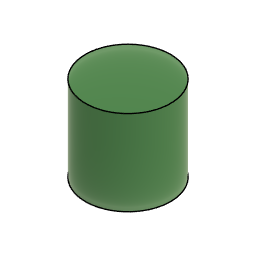
PE1-PE7 - PCB Enclosure Subassembly (Autodesk Fusion 360 archive; units mm, degrees)
design "Traceline Dummy"
Autodesk Fusion 360 part; units mm, degrees
note: some values were not read from the file. Chosen so that the rebuilt part matches the saved one: which bodies a step acts on; which face or edge a step refers to; the layout of a text. Set by a fixed rule: which sketch regions a step uses.
sketch "Sketch1" plane through (0, 0, 0) normal (0, 0, 1) x (1, 0, 0)
  circle A0 centre (0, 0) radius 0.05
  dimension "d1" = 0.1
  constraint coincident A0.centre origin
  measures "d1" diameter of A0
extrude "Extrude1" add sketch "Sketch1" along normal blind 0.1

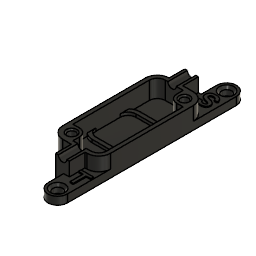
design "PE3 - PCB Case"
Autodesk Fusion 360 part; units mm, degrees
sketch "Sketch1" plane through (0, 0, 0) normal (0, 0, 1) x (1, 0, 0)
  line L0 (6.2013, 10.25) -> (-6.2012, 10.25)
  line L1 (-10.25, 6.2013) -> (-10.25, -6.2012)
  line L2 (-6.2012, -10.25) -> (6.2013, -10.25)
  line L3 (10.25, -6.2012) -> (10.25, 6.2012)
  line L4 (10.25, 10.25) -> (-10.25, -10.25) construction
  line L5 (-10.25, 10.25) -> (10.25, -10.25) construction
  arc A0 (-6.2012, 10.25) -> (-10.25, 6.2013) centre (-6.2013, 6.2013) ccw
  arc A1 (10.25, 6.2012) -> (6.2013, 10.25) centre (6.2012, 6.2012) ccw
  arc A2 (-10.25, -6.2012) -> (-6.2012, -10.25) centre (-6.2013, -6.2013) ccw
  arc A3 (6.2013, -10.25) -> (10.25, -6.2012) centre (6.2013, -6.2013) ccw
  line L6 (-12.25, 6.2013) -> (-12.25, -6.2013)
  arc A4 (-12.25, -6.2012) -> (-6.2012, -12.25) centre (-6.2013, -6.2013) ccw
  line L7 (-6.2012, -12.25) -> (6.2013, -12.25)
  arc A5 (6.2013, -12.25) -> (12.25, -6.2012) centre (6.2013, -6.2013) ccw
  line L8 (12.25, -6.2012) -> (12.25, 6.2012)
  arc A6 (12.25, 6.2012) -> (6.2013, 12.25) centre (6.2012, 6.2012) ccw
  line L9 (6.2013, 12.25) -> (-6.2012, 12.25)
  arc A7 (-6.2012, 12.25) -> (-12.25, 6.2013) centre (-6.2013, 6.2013) ccw
  dimension "d1" = 20.5
  dimension "d2" = 20.5
  dimension "d3" = 4.0488
  dimension "d4" = 4.0488
  dimension "d5" = 4.0488
  dimension "d6" = 4.0488
  dimension "d7" = 2
  constraint horizontal L0
  constraint perpendicular L0 L1
  constraint parallel L0 L2
  constraint parallel L1 L3
  constraint coincident L4 origin
  constraint coincident L5 origin
  constraint coincident L5.start L0
  constraint coincident L5.start L1
  constraint tangent L0 A0
  constraint tangent L1 A0
  constraint coincident L4.start L0
  constraint coincident L4.start L3
  constraint tangent L0 A1
  constraint tangent L3 A1
  constraint coincident L4.end L2
  constraint coincident L4.end L1
  constraint tangent L2 A2
  constraint tangent L1 A2
  constraint coincident L5.end L3
  constraint coincident L5.end L2
  constraint tangent L3 A3
  constraint tangent L2 A3
  measures "d1" distance of L4.start L5.start
  measures "d2" distance of L4.start L5.end
  measures "d3" radius of A0
  measures "d4" radius of A1
  measures "d5" radius of A2
  measures "d6" radius of A3
extrude "Extrude1" add sketch "Sketch1" along normal blind 6 contours L0 L1 L2 L3 A0 A1 A2 A3 | L6 A4 L7 A5 L8 A6 L9 A7
extrude "Extrude2" add sketch "Sketch1" along normal blind 1.5 from surface at 6
sketch "Sketch10" plane through (0, 0, 0) normal (0, 0, 1) x (1, 0, 0)
  line L0 (7.2501, -43.2789) -> (7.2501, 43.2211) construction
  line L1 (7.2501, -0.0289) -> (8.1135, -0.0289) construction
  circle A0 centre (7.2501, 43.2211) radius 2.5
  circle A1 centre (7.2501, -43.2789) radius 2.5
  arc A2 (2.2502, -43.2493) -> (12.25, -43.25) centre (7.2501, -43.2789) ccw
  arc A3 (12.25, 43.1922) -> (2.2502, 43.1914) centre (7.2501, 43.2211) ccw
  line L2 (2.2502, 43.1914) -> (2.2502, -43.3086)
  line L3 (12.25, -43.25) -> (12.25, 43.25)
  dimension "d42" = 86.5
  dimension "d43" = 5
  dimension "d44" = 5
  dimension "d45" = 10
  dimension "d46" = 10
  dimension "d134" = 0.0289
  dimension "d135" = 7.2501
  dimension "d136" = 0.8634
  constraint midpoint L0 L1.start
  constraint perpendicular L0 L1
  constraint coincident L0.end A0.centre
  constraint coincident L0.start A1.centre
  constraint concentric A1 A2
  constraint concentric A0 A3
  constraint parallel L0 L2
  constraint coincident A2 L2.end
  constraint coincident L2 A2.start
  constraint vertical L3
  constraint coincident L3 A3.start
  constraint coincident A3 L3.end
  constraint parallel L0 L3
  constraint equal L0 L2
  constraint equal L0 L3
  measures "d42" distance of L0.start L0.end
  measures "d43" diameter of A0
  measures "d44" diameter of A1
  measures "d45" diameter of A2
  measures "d46" diameter of A3
  measures "d134" distance of origin L1
  measures "d135" distance of origin L0
  measures "d136" distance of L0 L1.end
extrude "Extrude10" add sketch "Sketch10" along normal blind 4
chamfer "Chamfer1" distance 1.25 angle 45 2 edges at (6.346, -45.6097, 4) (6.346, 40.8903, 4)
sketch "Sketch12" plane through (0, 0, 0) normal (0, 0, -1) x (1, 0, 0)
  circle A0 centre (7.2501, 43.2789) radius 2.5
  circle A1 centre (7.2501, -43.2211) radius 2.5
  line L0 (2.2502, 12.25) -> (-6.2012, 12.25)
  arc A2 (-6.2013, 12.25) -> (-12.25, 6.2012) centre (-6.2013, 6.2013) ccw
  line L1 (-12.25, 6.2012) -> (-12.25, -6.2013)
  arc A3 (-12.25, -6.2013) -> (-6.2012, -12.25) centre (-6.2013, -6.2013) ccw
  line L2 (2.2502, -12.25) -> (2.2502, -43.1914)
  arc A4 (2.2502, -43.1914) -> (12.25, -43.25) centre (7.2501, -43.2211) ccw
  line L3 (12.25, -43.25) -> (12.25, 43.25)
  arc A5 (12.25, 43.25) -> (2.2502, 43.3086) centre (7.2501, 43.2789) ccw
  line L4 (10.25, -21.2012) -> (10.25, 21.2013)
  arc A6 (-6.2013, 25.25) -> (-10.25, 21.2013) centre (-6.2013, 21.2013) ccw
  arc A7 (-12.25, -21.2012) -> (-6.2013, -27.25) centre (-6.2013, -21.2012) ccw
  arc A8 (6.2013, -25.25) -> (10.25, -21.2012) centre (6.2013, -21.2012) ccw
  line L5 (-10.25, 25.25) -> (10.25, -25.25) construction
  line L6 (10.25, 25.25) -> (-10.25, -25.25) construction
  line L7 (-12.25, 21.2012) -> (-12.25, -21.2012)
  line L8 (-10.25, 21.2013) -> (-10.25, -21.2012)
  arc A9 (12.25, 21.2013) -> (6.2013, 27.25) centre (6.2012, 21.2013) ccw
  arc A10 (-6.2012, 27.25) -> (-12.25, 21.2012) centre (-6.2013, 21.2013) ccw
  line L9 (-6.2013, -25.25) -> (6.2013, -25.25)
  line L10 (6.2012, 25.25) -> (-6.2013, 25.25)
  line L11 (12.25, -21.2012) -> (12.25, 21.2013)
  arc A11 (10.25, 21.2013) -> (6.2012, 25.25) centre (6.2012, 21.2013) ccw
  arc A12 (-10.25, -21.2012) -> (-6.2013, -25.25) centre (-6.2013, -21.2012) ccw
  arc A13 (6.2012, -27.25) -> (12.25, -21.2012) centre (6.2013, -21.2012) ccw
  line L12 (-6.2013, -27.25) -> (6.2012, -27.25)
  line L13 (6.2013, 27.25) -> (-6.2012, 27.25)
  line L14 (-6.2012, -12.25) -> (2.2502, -12.25)
  line L15 (2.2502, 43.3086) -> (2.2502, 12.25)
  dimension "d77" = 2
  dimension "d78" = 20.5
  dimension "d79" = 50.5
  dimension "d80" = 4.0488
  dimension "d81" = 4.0488
  dimension "d82" = 4.0488
  dimension "d83" = 4.0488
  constraint horizontal L10
  constraint perpendicular L8 L10
  constraint parallel L9 L10
  constraint parallel L4 L8
  constraint coincident origin L6
  constraint coincident origin L5
  constraint coincident L5.start L10
  constraint coincident L5.start L8
  constraint tangent A6 L10
  constraint tangent A6 L8
  constraint coincident L6.start L10
  constraint coincident L6.start L4
  constraint tangent L10 A11
  constraint tangent L4 A11
  constraint coincident L6.end L9
  constraint coincident L6.end L8
  constraint tangent L9 A12
  constraint tangent L8 A12
  constraint coincident L5.end L4
  constraint coincident L5.end L9
  constraint tangent L4 A8
  constraint tangent A8 L9
  measures "d78" distance of L5.start L6.start
  measures "d79" distance of L5.end L6.start
  measures "d80" radius of A6
  measures "d81" radius of A11
  measures "d82" radius of A12
  measures "d83" radius of A8
extrude "Extrude13" cut 1 faces at (-3.4167, 2.0671, 6) along direction (0, 0, -1) blind 1
extrude "Extrude14" add sketch "Sketch12" against normal blind 11 contours L2 L3 L4 A8 A9 L9 L10 L11 A11 A13 L12 L13 L15 | A2 A6 L7 L8 A10 L10 L13 L15 | A2 L1 A3 L7 L8 | A3 L2 A7 L7 L8 L9 A12 L12
extrude "Extrude15" add sketch "Sketch12" against normal blind 4 contours L0 A2 A6 L8 L10 L15 | A3 L2 L8 L9 A12 L14
sketch "Sketch13" plane through (0, -27.25, 0) normal (0, -1, 0) x (1, 0, 0)
  line L0 (2.2502, 0) -> (2.2502, 4)
  line L1 (2.2502, 4) -> (6.2013, 4)
  line L2 (6.2013, 4) -> (6.2013, 11)
  line L3 (6.2013, 11) -> (-6.2012, 11)
  line L4 (-6.2012, 11) -> (-6.2012, 0)
  line L5 (-6.2012, 0) -> (2.2502, 0)
  line L6 (-1.8, 0) -> (5.2012, 0)
  line L7 (5.2012, 11) -> (5.2012, 0)
  line L8 (6.2012, 4) -> (3.0821, 4)
  line L9 (-1.8, 11) -> (-1.8, -1.0165)
  line L10 (-1.8, 0) -> (5.2012, 0)
  line L11 (-1.8, -1.0165) -> (-1.8, 0)
  line L12 (3.85, 11) -> (5.2012, 11)
  line L13 (-0.45, 11) -> (-1.8, 11)
  arc A0 (-0.45, 11) -> (3.85, 11) centre (1.7, 11) ccw
  point P0 (1.7, 11)
  dimension "d89" = 7
  dimension "d90" = 4.3
  constraint horizontal L10
  constraint horizontal L8
  constraint coincident P0 A0.centre
  constraint coincident L6.end L7.end
  constraint perpendicular L6 L7
  constraint perpendicular L10 L11
  constraint coincident L5 L6.start
  constraint perpendicular L7 L12
  constraint perpendicular L9 L13
  measures "d89" distance of L9.end L8.end
  measures "d90" diameter of A0
sketch "Sketch14" plane through (0, 27.25, 0) normal (0, 1, 0) x (-1, 0, 0)
  line L0 (-2.2502, 4) -> (-2.2502, 0)
  line L1 (-2.2502, 0) -> (6.2013, 0)
  line L2 (6.2013, 0) -> (6.2013, 11)
  line L3 (6.2013, 11) -> (-6.2012, 11)
  line L4 (-6.2012, 11) -> (-6.2012, 4)
  line L5 (-6.2012, 4) -> (-2.2502, 4)
  line L6 (-6.2013, 0) -> (-6.2013, 4)
  line L7 (-0.8, 15) -> (-0.8, 4)
  line L8 (-6.2013, 0) -> (6.2012, 0)
  line L9 (-0.8, 15) -> (6.2012, 15)
  line L10 (6.2012, 4) -> (6.2, 4)
  line L11 (6.2012, 15) -> (6.2012, 0)
  circle A0 centre (2.7, 11) radius 2.15
  line L12 (-0.8, 4) -> (-6.2013, 4)
  line L13 (-6.2013, 0) -> (6.2012, 0)
  point P0 (2.7, 11)
  dimension "d91" = 7
  dimension "d92" = 4.3
  dimension "d137" = 12.4012
  dimension "d138" = 7
  dimension "d139" = 11
  dimension "d140" = 0.0012
  dimension "d141" = 3.5
  constraint horizontal L13
  constraint horizontal L10
  constraint collinear L10 L12
  constraint coincident P0 A0.centre
  constraint coincident L8.end L11.end
  constraint perpendicular L8 L11
  constraint coincident L6.start L8.start
  constraint perpendicular L6 L12
  constraint coincident L4.end L6.end
  constraint perpendicular L7 L12
  constraint equal L0 L6
  constraint coincident L10.start L11
  constraint perpendicular L7 L9
  constraint coincident L1 origin
  measures "d91" distance of L7.end L10.end
  measures "d92" diameter of A0
  measures "d137" distance of L4 L10.end
  measures "d138" distance of L5 P0
  measures "d139" distance of L10.start L9
  measures "d140" distance of L10.end L11
  measures "d141" distance of P0 L7
extrude "Extrude16" add sketch "Sketch13" along normal blind 8 contours L0 L1 L3 L5 L6 L7 L8 L9 L10 L12 L13 A0
extrude "Extrude17" add sketch "Sketch13" along normal blind 8 contours L0 L1 L3 L5 L6 L7 L8 L9 L10 L12 L13 A0
extrude "Extrude18" add sketch "Sketch14" along normal blind 8 contours L0 L1 L2 L3 L7 L8 L11 A0 L12 L13
extrude "Extrude19" cut 1 faces at (-2.4382, 27.25, 10.3329) along direction (0, -1, 0) blind 5
extrude "Extrude20" cut 1 faces at (1.9618, -27.25, 10.3329) along direction (0, 1, 0) blind 4
sketch "Sketch15" plane through (0, 0, 4) normal (0, 0, 1) x (-1, 0, 0)
  line L0 (-10.25, 21.2013) -> (-10.25, 10.6951)
  arc A0 (-6.2013, 12.25) -> (-10.25, 10.6951) centre (-6.2013, 6.2013) ccw
  line L1 (-6.2013, 12.25) -> (6.2013, 12.25)
  arc A1 (10.25, 10.6951) -> (6.2012, 12.25) centre (6.2013, 6.2013) ccw
  line L2 (10.25, 10.6951) -> (10.25, 21.2013)
  arc A2 (10.25, 21.2013) -> (6.2013, 25.25) centre (6.2013, 21.2013) ccw
  line L3 (6.2013, 25.25) -> (-6.2012, 25.25)
  arc A3 (-6.2012, 25.25) -> (-10.25, 21.2013) centre (-6.2012, 21.2013) ccw
  circle A4 centre (6.9428, 21.9428) radius 2
  line L4 (8.8794, 25.9428) -> (2.9428, 25.9428)
  line L5 (2.9428, 25.9428) -> (2.9428, 21.9428)
  line L6 (6.9428, 17.9428) -> (10.9428, 17.9428)
  line L7 (10.9428, 17.9428) -> (10.9428, 23.8794)
  arc A5 (2.9428, 21.9428) -> (6.9428, 17.9428) centre (6.9428, 21.9428) ccw
  line L8 (10.9428, 17.9428) -> (10.9428, 23.8794)
  line L9 (8.8794, 25.9428) -> (2.9428, 25.9428)
  line L10 (2.9428, 25.9428) -> (2.9428, 21.9428)
  line L11 (6.9428, 17.9428) -> (10.9428, 17.9428)
  arc A6 (2.9428, 21.9428) -> (6.9428, 17.9428) centre (6.9428, 21.9428) ccw
  circle A7 centre (6.9428, 21.9428) radius 2
  line L12 (-1.75, 0) -> (-22.5, 0) construction
  line L13 (0, -2.5) -> (0, -20) construction
  line L14 (-8.0247, -25.9428) -> (-2.9428, -25.9428)
  line L15 (-2.9428, -25.9428) -> (-2.9428, -21.9428)
  arc A8 (-2.9428, -21.9428) -> (-6.9428, -17.9428) centre (-6.9428, -21.9428) ccw
  line L16 (-10.9428, -17.9428) -> (-10.9428, -23.0247)
  line L17 (-6.9428, -17.9428) -> (-10.9428, -17.9428)
  circle A9 centre (-6.9428, -21.9428) radius 2
  line L18 (-8.0247, -25.9428) -> (-10.9428, -23.0247)
  line L19 (-8.0247, -25.9428) -> (-3.8978, -25.9428) construction
  line L20 (10.9428, 23.8794) -> (8.8794, 25.9428)
  point P0 (6.9428, 21.9428)
  dimension "d106" = 4
  dimension "d109" = 4
  dimension "d114" = 4
  dimension "d115" = 4
  dimension "d116" = 135
  dimension "d142" = 17.9428
  dimension "d143" = 25.9428
  dimension "d144" = 23.0247
  dimension "d145" = 5.8857
  dimension "d149" = 23.8794
  dimension "d150" = 5.9366
  dimension "d151" = 17.9428
  dimension "d152" = 8
  constraint horizontal L4
  constraint perpendicular L4 L5
  constraint parallel L4 L6
  constraint parallel L5 L7
  constraint tangent L5 A5
  constraint tangent L6 A5
  constraint horizontal L9
  constraint perpendicular L9 L10
  constraint parallel L9 L11
  constraint parallel L8 L10
  constraint tangent L10 A6
  constraint tangent L11 A6
  constraint horizontal L19
  constraint tangent A8 L17
  constraint tangent L15 A8
  constraint concentric A8 A9
  constraint concentric A5 A7
  constraint equal A5 A8
  constraint midpoint A5 A6
  constraint equal L5 L10
  constraint equal L5 L11
  constraint equal L5 L15
  constraint equal L5 L17
  constraint perpendicular L16 L17
  constraint equal L18 L19
  constraint equal A4 A9
  constraint concentric A4 A5
  constraint coincident P0 A4.centre
  measures "d106" diameter of A4
  measures "d109" radius of A5
  measures "d114" diameter of A7
  measures "d115" radius of A6
  measures "d116" angle of L18 L19
  measures "d142" distance of L12 L17
  measures "d143" distance of L12 L19
  measures "d144" distance of L12 L16.end
  measures "d145" distance of L5 L15
  measures "d149" distance of L12 L7.end
  measures "d150" distance of L5 L4.start
  measures "d151" distance of L6 L12
  measures "d152" distance of L5 L7
extrude "Extrude21" add sketch "Sketch15" along normal blind 7 contours L2 A2 L3 L5 L6 A5 L10 L11 A6 | L14 L15 A8 L16 L17 L18
chamfer "Chamfer5" distance 0.7 angle 45 2 edges at (8.8075, 21.2196, 11) (-5.0782, -22.6661, 11)
extrude "Extrude24" cut 2 faces at (3.0992, -19.4386, 4) (-3.0992, 19.4386, 4) along direction (0, 0, -1) blind 2
extrude "Extrude25" cut 1 faces at (-3.4167, 2.0671, 5) along direction (0, 0, -1) blind 3
sketch "Sketch16" plane through (0, 0, 4) normal (0, 0, 1) x (-1, 0, 0)
  arc A0 (-12.25, -21.2012) -> (-6.2012, -27.25) centre (-6.2013, -21.2012) ccw
  line L0 (-12.25, -21.2012) -> (-12.25, -43.25)
  arc A1 (-12.25, -43.25) -> (-2.2502, -43.1914) centre (-7.2501, -43.2211) ccw
  line L1 (-2.2502, -43.1914) -> (-2.2502, -35.25)
  line L2 (-2.2502, -35.25) -> (-0.8, -35.25)
  line L3 (-0.8, -35.25) -> (-0.8, -27.25)
  line L4 (-10.7579, -32.3932) -> (-6.9514, -32.3932) construction
  line L5 (-6.9514, -32.3932) -> (-6.9514, -27.9161) construction
  line L6 (-6.9514, -27.9161) -> (-10.7579, -27.9161) construction
  line L7 (-10.7579, -27.9161) -> (-10.7579, -32.3932) construction
  line L8 (-0.8, -27.25) -> (-6.2012, -27.25)
  circle A2 centre (-7.2501, -43.2211) radius 3.75
  dimension "d124" = 8
  dimension "d153" = 5.2986
  dimension "d154" = 15.3339
  dimension "d155" = 3.8065
  dimension "d156" = 4.4771
  text T0 "S" font "Arial" height 8 bold align left top in box 3.8065 x 4.4771 at (-10.7579, -32.3932) x (1, 0) y (0, 1) spacing 1 by line height
  measures "d153" distance of L0 L5
  measures "d154" distance of L0.end L6
  measures "d155" distance of L5 L7
  measures "d156" distance of L4 L6
extrude "Extrude26" add sketch "Sketch16" along normal blind 0.5 text T0
sketch "Sketch17" plane through (0, 0, 4) normal (0, 0, 1) x (-1, 0, 0)
  circle A0 centre (-7.2501, 43.2789) radius 3.75
  line L0 (-5.2012, 27.25) -> (-5.2012, 35.25)
  line L1 (-5.2012, 35.25) -> (-2.2502, 35.25)
  line L2 (-2.2502, 35.25) -> (-2.2502, 43.3086)
  arc A1 (-2.2502, 43.3086) -> (-12.25, 43.25) centre (-7.2501, 43.2789) ccw
  line L3 (-12.25, 43.25) -> (-12.25, 21.2013)
  arc A2 (-6.2013, 27.25) -> (-12.25, 21.2013) centre (-6.2012, 21.2013) ccw
  line L4 (-6.2013, 27.25) -> (-5.2012, 27.25)
  line L5 (-5.3111, 31.9604) -> (-9.1175, 31.9604) construction
  line L6 (-9.1175, 31.9604) -> (-9.1175, 27.4833) construction
  line L7 (-9.1175, 27.4833) -> (-5.3111, 27.4833) construction
  line L8 (-5.3111, 27.4833) -> (-5.3111, 31.9604) construction
  dimension "d127" = 8
  dimension "d157" = 6.9389
  dimension "d158" = 6.282
  dimension "d159" = 4.4771
  dimension "d160" = 3.8065
  text T0 "T" font "Arial" height 8 bold align left top in box 3.8065 x 4.4771 at (-5.3111, 31.9604) x (-1, 0) y (0, -1) spacing 1 by line height
  constraint vertical L8
  measures "d157" distance of L3 L8
  measures "d158" distance of L3.end L7
  measures "d159" distance of L5 L7
  measures "d160" distance of L6 L8
extrude "Extrude27" add sketch "Sketch17" along normal blind 0.5 text T0
extrude "Extrude28" cut 2 faces at (-2.0671, 10.9167, 7.5) (-2.0671, -11.5833, 7.5) along direction (0, 0, -1) blind 4
equation "d3 = ( 20.5 / 20 * 3.95 ) * 1 mm"
equation "d4 = ( 20.5 / 20 * 3.95 ) * 1 mm"
equation "d5 = ( 20.5 / 20 * 3.95 ) * 1 mm"
equation "d6 = ( 20.5 / 20 * 3.95 ) * 1 mm"
equation "d80 = ( 20.5 / 20 * 3.95 ) * 1 mm"
equation "d81 = ( 20.5 / 20 * 3.95 ) * 1 mm"
equation "d82 = ( 20.5 / 20 * 3.95 ) * 1 mm"
equation "d83 = ( 20.5 / 20 * 3.95 ) * 1 mm"

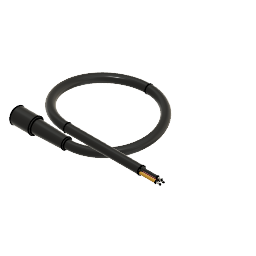
design "PE2 - 3-Pin Male Waterproof Connector (coiled)"
Autodesk Fusion 360 part; units mm, degrees
sketch "Sketch1" plane through (0, 0, 0) normal (1, 0, 0) x (0, 1, 0)
  circle A0 centre (0, 0) radius 3.683
  circle A1 centre (0, 0) radius 3.175
  dimension "d1" = 7.366
  dimension "d2" = 6.35
  constraint coincident A0.centre A1.centre
  constraint concentric A0 A1
  measures "d1" diameter of A0
  measures "d2" diameter of A1
extrude "Extrude1" add sketch "Sketch1" along normal blind 10 contours A0 | A1 makes body 1
extrude "Extrude2" cut sketch "Sketch1" along normal blind 8 contours A1 bodies 1
sketch "Sketch2" plane through (0, 0, 0) normal (0, 1, 0) x (1, 0, 0)
  line L0 (10, 0) -> (10, -3)
  line L1 (10, -3) -> (25, -2.5)
  line L2 (25, -2.5) -> (25, 0)
  line L3 (25, 0) -> (10, 0)
  dimension "d7" = 3
  dimension "d44" = 15
  dimension "d45" = 88.091
  dimension "d46" = 10
  constraint vertical L0
  constraint vertical L2
  constraint perpendicular L0 L3
  constraint horizontal origin L0.start
  measures "d7" distance of L0.start L0.end
  measures "d44" distance of L0 L2
  measures "d45" angle of L0 L1
  measures "d46" distance of origin L0
revolve "Revolve1" add sketch "Sketch2" angle 360 about axis through (1.75, 0, 0) along (1, 0, 0) bodies 1
fillet "Fillet1" radius 0.5 3 edges at (0, -3.4338, -1.3318) (10, -3.4338, -1.3318) (25, -0.904, -2.3308) on bodies 1
sketch "Sketch4" plane through (8, 0, 0) normal (1, 0, 0) x (0, 1, 0)
  line L0 (0, 1.5) -> (-1.299, -0.75) construction
  line L1 (-1.299, -0.75) -> (1.299, -0.75) construction
  line L2 (1.299, -0.75) -> (0, 1.5) construction
  circle A0 centre (0, 1.5) radius 0.5
  circle A1 centre (-1.299, -0.75) radius 0.5
  circle A2 centre (1.299, -0.75) radius 0.5
  dimension "d15" = 1.5
  dimension "d16" = 1
  dimension "d17" = 1
  dimension "d18" = 1
  constraint coincident L0.start L2.end
  constraint coincident L0.end L1.start
  constraint coincident L1.end L2.start
  constraint horizontal L1
  measures "d15" distance of L0.start origin
  measures "d16" diameter of A0
  measures "d17" diameter of A1
  measures "d18" diameter of A2
extrude "Extrude4" add sketch "Sketch4" against normal blind 8 separate body makes body 2 at (2.6667, 0.4975, 1.4502) makes body 3 at (2.6667, 1.7966, -0.7998) makes body 4 at (2.6667, -0.8015, -0.7998)
fillet "Fillet2" radius 0.1 3 edges at (0, -0.4662, 1.6808) (0, 0.8329, -0.5692) (0, -1.7652, -0.5692) on bodies 2 3 4
sketch "Sketch3" plane through (25, 0, 0) normal (1, 0, 0) x (0, 1, 0)
  circle A0 centre (0, 0) radius 1.905
  circle A1 centre (0, 0) radius 2.0164
  dimension "d9" = 3.81
  constraint coincident A0.centre A1.centre
  measures "d9" diameter of A0
sketch "Sketch5" plane through (0, 0, 0) normal (0, 0, 1) x (1, 0, 0)
  arc A0 through (25, 0, 0) (45, 19.9239, 1.7431) (25, 39.8478, 3.4862)
  arc A1 through (25, 39.8478, 3.4862) (5, 19.9239, 5.2293) (25, 0, 6.9725)
  dimension "d42" = 40
  dimension "d47" = 20
  dimension "d48" = 3.4862
  dimension "d49" = 6.9725
sweep "Sweep1" add profiles "Sketch3" path "Sketch5" along A0 A1 section 1 contours A0 bodies 1
extrude "Extrude5" add 1 faces at (25, -0.7992, 7.2336) along direction (1, 0, 0) blind 36.2 on bodies 1 bodies 1
sketch "Sketch6" plane through (61.2, 0, 0) normal (1, 0, 0) x (0, 1, 0)
  line L0 (0, 7.9725) -> (-0.866, 6.4725) construction
  line L1 (-0.866, 6.4725) -> (0.866, 6.4725) construction
  line L2 (0.866, 6.4725) -> (0, 7.9725) construction
  circle A0 centre (0, 7.9725) radius 0.625
  circle A1 centre (0.866, 6.4725) radius 0.625
  circle A2 centre (-0.866, 6.4725) radius 0.625
  circle A3 centre (0, 6.9725) radius 1.905
  point P0 (0, 6.9725)
  dimension "d31" = 1
  dimension "d32" = 1.25
  dimension "d33" = 1.25
  dimension "d34" = 1.25
  constraint coincident L0.start L2.end
  constraint coincident L1.end L2.start
  constraint coincident L0.end L1.start
  constraint coincident P0 A3.centre
  constraint vertical L0.start P0
  measures "d31" distance of L0.start P0
  measures "d32" diameter of A0
  measures "d33" diameter of A1
  measures "d34" diameter of A2
extrude "Extrude6" add sketch "Sketch6" along normal blind 8 separate body contours A0 | A1 | A2 makes body 5 at (63.8667, 0.6219, 7.9102) makes body 6 at (63.8667, -0.2441, 6.4102) makes body 7 at (63.8667, 1.4879, 6.4102)
sketch "Sketch7" plane through (69.2, 0, 0) normal (1, 0, 0) x (0, 1, 0)
  circle A0 centre (0, 7.9725) radius 0.625
  circle A1 centre (0, 7.9725) radius 0.375
  dimension "d43" = 0.75
  constraint concentric A0 A1
  measures "d43" diameter of A1
sketch "Sketch8" plane through (69.2, 0, 0) normal (1, 0, 0) x (0, 1, 0)
  circle A0 centre (0.866, 6.4725) radius 0.625
  circle A1 centre (0.866, 6.4725) radius 0.375
  dimension "d37" = 0.75
  constraint concentric A0 A1
  measures "d37" diameter of A1
sketch "Sketch9" plane through (69.2, 0, 0) normal (1, 0, 0) x (0, 1, 0)
  circle A0 centre (-0.866, 6.4725) radius 0.625
  circle A1 centre (-0.866, 6.4725) radius 0.375
  dimension "d38" = 0.75
  constraint concentric A0 A1
  measures "d38" diameter of A1
extrude "Extrude7" add sketch "Sketch9" sketch "Sketch8" sketch "Sketch7" along normal blind 2 separate body contours A1 of sketch 2 contours A1 of sketch 3 contours A1 makes body 8 at (69.8667, 1.2392, 6.4351) makes body 9 at (69.8667, -0.4929, 6.4351) makes body 10 at (70.5333, -0.3524, 8.1007)

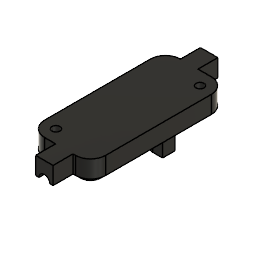
design "PE4 - PCB Case Lid"
Autodesk Fusion 360 part; units mm, degrees
sketch "Sketch1" plane through (0, 0, 0) normal (0, 0, 1) x (1, 0, 0)
  line L0 (6.2013, 11.75) -> (-6.2012, 11.75)
  line L1 (10.25, 10.25) -> (-10.25, -10.25) construction
  arc A0 (-6.2012, 11.75) -> (-11.75, 6.2013) centre (-6.2013, 6.2013) ccw
  line L2 (-11.75, 6.2013) -> (-11.75, -6.2013)
  arc A1 (-11.75, -6.2012) -> (-6.2012, -11.75) centre (-6.2013, -6.2013) ccw
  line L3 (-6.2012, -11.75) -> (6.2013, -11.75)
  arc A2 (11.75, 6.2012) -> (6.2013, 11.75) centre (6.2012, 6.2012) ccw
  arc A3 (6.2013, -11.75) -> (11.75, -6.2012) centre (6.2013, -6.2013) ccw
  line L4 (-10.25, 10.25) -> (10.25, -10.25) construction
  line L5 (11.75, -6.2012) -> (11.75, 6.2012)
  circle A4 centre (6.2012, 6.2012) radius 1.7
  circle A5 centre (-6.2013, -6.2013) radius 1.7
  line L6 (-6.2013, -6.2013) -> (-6.2013, -4) construction
  line L7 (-6.2013, -6.2013) -> (-4, -6.2013) construction
  line L8 (-4, -6.2013) -> (-4, -10.15)
  line L9 (-6.2013, -4) -> (-10.15, -4)
  line L10 (-4, -6.2013) -> (-4, -5)
  line L11 (-6.2013, -4) -> (-5, -4)
  arc A6 (-4, -5) -> (-5, -4) centre (-5, -5) ccw
  line L12 (6.2013, 4) -> (10.15, 4)
  line L13 (6.2013, 4) -> (5, 4)
  arc A7 (4, 5) -> (5, 4) centre (5, 5) ccw
  line L14 (4, 6.2013) -> (4, 5)
  line L15 (4, 6.2013) -> (4, 10.15)
  line L16 (10.15, -6.2012) -> (10.15, 6.2012)
  arc A8 (10.15, 6.2012) -> (6.2013, 10.15) centre (6.2012, 6.2012) ccw
  line L17 (6.2012, 10.15) -> (-6.2012, 10.15)
  arc A9 (-6.2012, 10.15) -> (-10.15, 6.2013) centre (-6.2013, 6.2013) ccw
  line L18 (-10.15, 6.2013) -> (-10.15, -6.2012)
  arc A10 (-10.15, -6.2012) -> (-6.2012, -10.15) centre (-6.2013, -6.2013) ccw
  line L19 (-6.2012, -10.15) -> (6.2013, -10.15)
  arc A11 (6.2013, -10.15) -> (10.15, -6.2013) centre (6.2013, -6.2013) ccw
  arc A12 (9.15, 6.2012) -> (6.2012, 9.15) centre (6.2012, 6.2012) ccw
  line L20 (6.2012, 9.15) -> (-6.2012, 9.15)
  arc A13 (-6.2012, 9.15) -> (-9.15, 6.2013) centre (-6.2013, 6.2013) ccw
  line L21 (-9.15, 6.2013) -> (-9.15, -6.2012)
  arc A14 (-9.15, -6.2012) -> (-6.2013, -9.15) centre (-6.2013, -6.2013) ccw
  line L22 (-6.2013, -9.15) -> (6.2013, -9.15)
  arc A15 (6.2013, -9.15) -> (9.15, -6.2013) centre (6.2013, -6.2013) ccw
  line L23 (9.15, -6.2013) -> (9.15, 6.2012)
  dimension "d2" = 20.5
  dimension "d3" = 20.5
  dimension "d8" = 3.4
  dimension "d9" = 3.4
  dimension "d13" = 1
  dimension "d26" = -1.6
  dimension "d27" = -2.6
  dimension "d89" = 5
  dimension "d90" = 9
  dimension "d91" = 9
  dimension "d92" = 6.75
  dimension "d93" = 1.2012
  dimension "d94" = 1
  dimension "d95" = 14.15
  dimension "d96" = 6.75
  dimension "d97" = 1.2012
  dimension "d98" = 14.15
  dimension "d99" = 2.2012
  dimension "d100" = 2.2012
  dimension "d101" = 2.2012
  dimension "d102" = 2.2012
  dimension "d103" = 135
  dimension "d104" = 5
  constraint coincident origin L1
  constraint coincident origin L4
  constraint vertical L6
  constraint perpendicular L6 L7
  constraint perpendicular L6 L9
  constraint perpendicular L7 L10
  constraint perpendicular L10 L11
  constraint tangent L10 A6
  constraint tangent L11 A6
  constraint vertical L15
  constraint horizontal L12
  constraint coincident L8.end L19
  constraint perpendicular L8 L19
  constraint coincident L9.end L18
  constraint perpendicular L9 L18
  constraint coincident L15.end L17
  constraint perpendicular L15 L17
  constraint coincident L12.end L16
  constraint perpendicular L12 L16
  constraint tangent A7 L14
  constraint tangent L13 A7
  constraint equal A6 A7
  constraint tangent A0 L2
  constraint tangent L0 A0
  constraint equal A0 A1
  constraint equal A0 A2
  constraint equal A0 A3
  constraint equal L10 L13
  constraint equal L10 L14
  constraint parallel L14 L15
  constraint parallel L12 L13
  constraint vertical L12.start L22.end
  constraint horizontal L14.start A12.start
  constraint midpoint origin L1
  constraint tangent L2 A1
  constraint equal L0 L2
  constraint equal L0 L18
  constraint equal L0 L21
  constraint equal L6 L7
  constraint equal L0 L23
  constraint equal L0 L16
  constraint equal L0 L5
  constraint tangent A1 L3
  constraint equal L0 L3
  constraint equal L0 L19
  constraint equal L0 L22
  constraint concentric A2 A4
  constraint concentric A1 A5
  constraint vertical L1.end L4.start
  constraint vertical L1.start L4.end
  constraint coincident A1.centre A5.centre
  measures "d2" distance of L1.start L4.start
  measures "d3" distance of L1.start L4.end
  measures "d8" diameter of A4
  measures "d9" diameter of A5
  measures "d13" radius of A6
  measures "d89" horizontal distance of origin A6.centre
  measures "d90" distance of A6.centre L13
  measures "d91" distance of A6.centre L14
  measures "d92" distance of L2 A6.centre
  measures "d93" distance of L6 A6.centre
  measures "d94" distance of L8 A6.centre
  measures "d95" distance of A6.centre L23
  measures "d96" distance of L3 A6.centre
  measures "d97" distance of L7 A6.centre
  measures "d98" distance of A6.centre L20
  measures "d99" distance of A0.centre L10
  measures "d100" distance of A3.centre L11
  measures "d101" distance of A2.centre L14
  measures "d102" distance of A2.centre L12
  measures "d103" angle of L1 L9
  measures "d104" vertical distance of origin A6.centre
sketch "Sketch2" plane through (0, 0, 0) normal (0, 0, 1) x (1, 0, 0)
  line L0 (-6.2013, -27.25) -> (6.2012, -27.25)
  arc A0 (6.2012, -27.25) -> (12.25, -21.2012) centre (6.2013, -21.2012) ccw
  line L1 (12.25, -21.2012) -> (12.25, 21.2013)
  arc A1 (12.25, 21.2013) -> (6.2013, 27.25) centre (6.2012, 21.2013) ccw
  line L2 (6.2013, 27.25) -> (-6.2012, 27.25)
  arc A2 (-6.2012, 27.25) -> (-12.25, 21.2013) centre (-6.2013, 21.2013) ccw
  line L3 (-12.25, 21.2013) -> (-12.25, -21.2012)
  arc A3 (-12.25, -21.2012) -> (-6.2013, -27.25) centre (-6.2013, -21.2012) ccw
  line L4 (-10.15, 21.2013) -> (-10.15, -21.2012)
  arc A4 (-10.15, -21.2012) -> (-6.2013, -25.15) centre (-6.2013, -21.2012) ccw
  line L5 (-6.2013, -25.15) -> (6.2013, -25.15)
  arc A5 (6.2013, -25.15) -> (10.15, -21.2012) centre (6.2013, -21.2012) ccw
  line L6 (10.15, -21.2012) -> (10.15, 17.8428)
  line L7 (2.8428, 25.15) -> (-6.2013, 25.15)
  arc A6 (-6.2013, 25.15) -> (-10.15, 21.2013) centre (-6.2013, 21.2013) ccw
  circle A7 centre (6.9428, 21.9428) radius 1.6
  circle A8 centre (-6.9428, -21.9428) radius 1.6
  line L8 (-6.2013, -25.15) -> (6.2012, -25.15)
  arc A9 (6.2012, -25.15) -> (10.15, -21.2012) centre (6.2013, -21.2012) ccw
  line L9 (10.15, -21.2012) -> (10.15, 21.2013)
  arc A10 (10.15, 21.2013) -> (6.2013, 25.15) centre (6.2012, 21.2013) ccw
  line L10 (6.2013, 25.15) -> (-6.2012, 25.15)
  arc A11 (-6.2012, 25.15) -> (-10.15, 21.2013) centre (-6.2013, 21.2013) ccw
  line L11 (-10.15, 21.2013) -> (-10.15, -21.2012)
  arc A12 (-10.15, -21.2012) -> (-6.2013, -25.15) centre (-6.2013, -21.2012) ccw
  line L12 (2.8428, 23.65) -> (-6.2013, 23.65)
  arc A13 (-6.2013, 23.65) -> (-8.65, 21.2013) centre (-6.2013, 21.2013) ccw
  line L13 (-8.65, 21.2013) -> (-8.65, -17.8428)
  line L14 (2.8428, 25.15) -> (2.8428, 23.65)
  line L15 (-8.65, -17.8428) -> (-10.15, -17.8428)
  line L16 (-2.8428, -23.65) -> (6.2013, -23.65)
  arc A14 (6.2013, -23.65) -> (8.65, -21.2012) centre (6.2013, -21.2012) ccw
  line L17 (8.65, -21.2012) -> (8.65, 17.8428)
  line L18 (-2.8428, -25.15) -> (-2.8428, -23.65)
  line L19 (10.15, 17.8428) -> (8.65, 17.8428)
  dimension "d62" = 3.2
  dimension "d63" = 3.2
  dimension "d71" = -2.1
  dimension "d105" = 8.65
  dimension "d106" = 17.8428
  dimension "d107" = 1.7072
  dimension "d108" = 15.5928
  dimension "d109" = 4.1
  dimension "d110" = 39.7857
  dimension "d111" = 6.0488
  dimension "d112" = 1.5
  dimension "d113" = 39.0441
  dimension "d114" = 2.4487
  dimension "d115" = 2.4488
  dimension "d116" = 5.8072
  dimension "d117" = 11.4928
  dimension "d118" = 14.8513
  dimension "d119" = 17.3
  dimension "d120" = 18.8
  dimension "d121" = 9.4072
  dimension "d122" = 5.8072
  dimension "d123" = 35.6857
  dimension "d124" = 7.3072
  dimension "d125" = 22.4
  dimension "d126" = 1.5
  constraint coincident L5 L18.start
  constraint perpendicular L7 L14
  constraint perpendicular L11 L15
  constraint coincident L4 L15.end
  constraint perpendicular L16 L18
  constraint perpendicular L17 L19
  constraint tangent A14 L17
  constraint tangent A13 L13
  constraint tangent L7 A11
  constraint tangent L3 A3
  constraint tangent L0 A3
  constraint tangent A2 L3
  constraint tangent L2 A2
  constraint tangent A1 L2
  constraint tangent L1 A1
  constraint tangent L0 A0
  constraint tangent A0 L1
  constraint concentric A6 A11
  constraint concentric A11 A13
  constraint concentric A3 A4
  constraint concentric A0 A5
  constraint coincident L4.start A11
  constraint perpendicular L13 L15
  constraint perpendicular L4 L15
  constraint equal A0 A3
  constraint equal A0 A2
  constraint equal A0 A1
  constraint equal L6 L13
  constraint equal L14 L15
  constraint midpoint A6 A11
  constraint midpoint L4 L11
  constraint parallel L0 L12
  constraint equal L7 L16
  measures "d62" diameter of A7
  measures "d63" diameter of A8
  measures "d105" distance of origin L13
  measures "d106" distance of origin L15
  measures "d107" distance of A8.centre L13
  measures "d108" distance of A7.centre L13
  measures "d109" distance of A8.centre L15
  measures "d110" distance of A7.centre L15
  measures "d111" radius of A2
  measures "d112" distance of L4.start L13
  measures "d113" distance of L1.end L15
  measures "d114" distance of L0.start L13
  measures "d115" distance of L2.end L13
  measures "d116" distance of L13 L18
  measures "d117" distance of L13 L14
  measures "d118" distance of A1.end L13
  measures "d119" distance of L13 L17
  measures "d120" distance of L9 L13
  measures "d121" distance of L0 L15
  measures "d122" distance of L15 L16
  measures "d123" distance of L15 L19
  measures "d124" distance of L18.start L15
  measures "d125" distance of L3 L6
  measures "d126" distance of A5 A14
extrude "Extrude5" add sketch "Sketch2" along normal blind 5 contours L0 A0 L1 A1 L2 A2 L3 A3 | L4 L7 A6 L10 A11 L11 L12 A13 L13 L14 L15 | L4 A4 L5 L8 L9 A10 L10 L11 A12 L12 A13 L13 L14 L15 L16 A14 L17 L18 L19 | L5 A5 L6 L8 A9 L9 L16 A14 L17 L18 L19 | A7 | A8
extrude "Extrude6" add sketch "Sketch2" against normal blind 2 contours L4 L7 A6 L10 A11 L11 L12 A13 L13 L14 L15 | L5 A5 L6 L8 A9 L9 L16 A14 L17 L18 L19
sketch "Sketch3" plane through (0, 0, 0) normal (0, 1, 0) x (1, 0, 0)
  line L0 (1.7, 3) -> (1.7, 0) construction
  line L1 (-0.45, 0) -> (-0.45, 2.15)
  line L2 (3.85, -0.0044) -> (3.85, 2.1456)
  line L3 (-0.45, 2.15) -> (3.85, 2.1456)
  arc A0 (1.7991, 2.1477) -> (1.6052, 2.1479) centre (1.7, 0) ccw
  arc A1 (-0.45, 0) -> (3.85, 0.0044) centre (1.7, 0) ccw
  line L4 (5.2, -5) -> (-1.8, -5)
  line L5 (-1.8, -5) -> (-1.8, 0)
  line L6 (5.2, 0) -> (5.2, -5)
  line L7 (5.2, -5) -> (0.1955, 2.1493) construction
  line L8 (-1.8, -5) -> (3.2024, 2.1463) construction
  line L9 (5.2, 0) -> (3.85, 0)
  line L10 (-0.45, 0) -> (-1.8, 0)
  point P0 (1.7, 0)
  dimension "d45" = 2.15
  dimension "d46" = 2.15
  dimension "d127" = 2.15
  dimension "d128" = 3.5
  dimension "d129" = 3.5
  dimension "d130" = 2.15
  dimension "d131" = 1.5045
  dimension "d132" = 1.5024
  dimension "d133" = 0.45
  dimension "d134" = 8
  constraint vertical L0
  constraint coincident L1.start A0
  constraint vertical L1
  constraint coincident L2.start A0
  constraint vertical L2
  constraint coincident L2 A1.end
  constraint coincident L3 A0.start
  constraint coincident L3 A0.end
  constraint concentric A0 A1
  constraint horizontal L4
  constraint perpendicular L4 L5
  constraint parallel L5 L6
  constraint coincident L7 P0
  constraint coincident L8 P0
  constraint coincident P0 L0.end
  constraint horizontal L9
  constraint coincident L3 L8.end
  constraint coincident L3 L7.end
  constraint coincident L2 L9.end
  constraint collinear L9 L10
  constraint horizontal origin L1.start
  constraint tangent L1 A1
  measures "d45" distance of L1.start L1.end
  measures "d46" distance of L2.start L2.end
  measures "d127" radius of A1
  measures "d128" distance of L0 L5
  measures "d129" distance of L0 L6
  measures "d130" distance of L0 L2
  measures "d131" distance of L0 L7.end
  measures "d132" distance of L0 L8.end
  measures "d133" distance of origin L1
  measures "d134" distance of L0.start L4
extrude "Extrude7" cut sketch "Sketch2" along normal blind 3 contours L4 A4 L5 L8 L9 A10 L10 L11 A12 L12 A13 L13 L14 L15 L16 A14 L17 L18 L19 | A7 | A8
extrude "Extrude8" cut sketch "Sketch3" against normal blind 31 contours L1 L2 L3 A0 A1
extrude "Extrude9" add sketch "Sketch3" against normal blind 8 from surface at -27.25 contours L2 A1 L4 L5 L6 L9 L10
sketch "Sketch4" plane through (0, 0, 0) normal (0, 1, 0) x (1, 0, 0)
  line L0 (6.2012, 4) -> (6.2, 4)
  line L1 (-6.2013, 0) -> (0.8, 0)
  line L2 (-4.85, 0) -> (-4.85, 2.15)
  line L3 (-4.85, 2.15) -> (-0.55, 2.1456)
  line L4 (-0.55, -0.0044) -> (-0.55, 2.1456)
  line L5 (-4.85, 0) -> (-2.7, 0) construction
  arc A0 (-4.85, 0) -> (-0.55, 0.0044) centre (-2.7, 0) ccw
  arc A1 (-2.6009, 2.1477) -> (-2.7948, 2.1479) centre (-2.7, 0) ccw
  line L6 (-6.2, -5) -> (0.8, -5)
  line L7 (0.8, -5) -> (0.8, 0)
  line L8 (-6.2, 0) -> (-6.2, -5)
  line L9 (-6.2, -5) -> (-1.1976, 2.1463) construction
  line L10 (0.8, -5) -> (-4.2045, 2.1493) construction
  line L11 (-4.85, 0) -> (-6.2013, 0)
  line L12 (-0.55, -0.0044) -> (0.8, 0)
  point P0 (-2.7, 0)
  dimension "d53" = 2.15
  dimension "d54" = 2.15
  dimension "d55" = 2.15
  dimension "d135" = 0.55
  dimension "d136" = 6.75
  dimension "d137" = 2.15
  dimension "d138" = 0.0044
  dimension "d139" = 1.35
  dimension "d140" = 4.9956
  dimension "d141" = 5.65
  dimension "d142" = 6.7513
  dimension "d143" = 4
  dimension "d144" = 5.6512
  constraint horizontal L1
  constraint horizontal L0
  constraint vertical L2
  constraint vertical L4
  constraint perpendicular L2 L5
  constraint coincident L3 A1.end
  constraint coincident L4 A0.end
  constraint coincident L3 A1.start
  constraint concentric A0 A1
  constraint horizontal L6
  constraint perpendicular L6 L7
  constraint parallel L7 L8
  constraint coincident L9 P0
  constraint coincident L10 P0
  constraint coincident P0 L5.end
  constraint perpendicular L8 L11
  constraint coincident L3 L9.end
  constraint coincident L3 L10.end
  constraint coincident L1 L8.start
  constraint tangent L2 A0
  constraint coincident L4.start A0
  constraint equal A0 A1
  constraint coincident origin L1
  measures "d53" distance of L2.start L2.end
  measures "d54" distance of L3.end L4.start
  measures "d55" distance of L2.start P0
  measures "d135" distance of origin L4
  measures "d136" distance of L0.end L4
  measures "d137" radius of A0
  measures "d138" distance of L4.start L5
  measures "d139" distance of L4 L7
  measures "d140" distance of L4.start L6
  measures "d141" distance of L4 L8
  measures "d142" distance of L0.start L4
  measures "d143" distance of L0 L11
  measures "d144" distance of L1.start L4
extrude "Extrude10" add sketch "Sketch4" along normal blind 8 from surface at 27.25 contours L1 A0 L6 L7 L8 L11 L12
extrude "Extrude11" cut sketch "Sketch4" along normal blind 61 contours L1 L2 L3 L4 A0 A1 | L1 L4 A0
extrude "Extrude12" cut sketch "Sketch2" along normal blind 20 contours A7 | A8
extrude "Extrude13" add 1 faces at (-4.3101, 7.137, 5) along direction (0, 0, 1) blind 2
sketch "Sketch5" plane through (0, 0, 3) normal (0, 0, -1) x (1, 0, 0)
  circle A0 centre (6.9428, -21.9428) radius 1.6
  circle A1 centre (-6.9428, 21.9428) radius 1.6
  arc A2 (-6.2013, 25.15) -> (-10.15, 21.2012) centre (-6.2013, 21.2012) ccw
  line L0 (-10.15, 21.2012) -> (-10.15, 17.8428)
  line L1 (2.8428, -25.15) -> (6.2013, -25.15)
  arc A3 (6.2013, -25.15) -> (10.15, -21.2013) centre (6.2012, -21.2013) ccw
  line L2 (10.15, -21.2013) -> (10.15, -17.8428)
  line L3 (9.15, -17.8428) -> (-9.15, -17.8428)
  line L4 (-9.15, -17.8428) -> (-9.15, 17.8428)
  line L5 (-9.15, 17.8428) -> (9.15, 17.8428)
  line L6 (9.15, 17.8428) -> (9.15, -17.8428)
  line L7 (-10.15, 17.8428) -> (-8.65, 17.8428)
  line L8 (-8.65, 17.8428) -> (-8.65, -21.2013)
  arc A4 (-8.65, -21.2013) -> (-6.2013, -23.65) centre (-6.2013, -21.2013) ccw
  line L9 (-6.2013, -23.65) -> (2.8428, -23.65)
  line L10 (2.8428, -23.65) -> (2.8428, -25.15)
  line L11 (10.15, -17.8428) -> (8.65, -17.8428)
  line L12 (8.65, -17.8428) -> (8.65, 21.2012)
  arc A5 (8.65, 21.2012) -> (6.2013, 23.65) centre (6.2013, 21.2012) ccw
  line L13 (6.2013, 23.65) -> (-2.8428, 23.65)
  line L14 (-2.8428, 23.65) -> (-2.8428, 25.15)
  line L15 (-2.8428, 25.15) -> (-6.2013, 25.15)
  dimension "d145" = 1
  dimension "d146" = 18.3
  constraint horizontal L3
  constraint vertical L4
  constraint horizontal L5
  constraint vertical L6
  constraint coincident L3.start L11
  constraint coincident L4.end L7
  measures "d145" distance of L0.end L4
  measures "d146" distance of L4 L6
extrude "Extrude14" cut sketch "Sketch5" against normal blind 2 contours L3 L4 L5 L7 L8 | L3 L5 L8 L12 | L3 L5 L6 L11 L12
sketch "Sketch6" plane through (0, 0, 5) normal (0, 0, -1) x (1, 0, 0)
  line L0 (9.15, 17.8428) -> (-9.15, 17.8428)
  line L1 (-9.15, 17.8428) -> (-9.15, -17.8428)
  line L2 (-9.15, -17.8428) -> (9.15, -17.8428)
  line L3 (9.15, -17.8428) -> (9.15, 17.8428)
  line L4 (6.2012, -6.2012) -> (6.2012, -3.7012) construction
  line L5 (6.2012, -3.7012) -> (9.15, -3.7012)
  line L6 (9.15, -8.7012) -> (6.2012, -8.7012)
  arc A0 (6.2012, -3.7012) -> (6.2012, -8.7012) centre (6.2012, -6.2012) ccw
  line L7 (-6.2013, 3.7013) -> (-9.15, 3.7013)
  line L8 (-9.15, 8.7013) -> (-6.2013, 8.7013)
  arc A1 (-6.2013, 3.7013) -> (-6.2013, 8.7013) centre (-6.2013, 6.2013) ccw
  line L9 (-9.15, 3.7013) -> (-10.15, 3.7013)
  line L10 (-10.15, 3.7013) -> (-10.15, 8.7013)
  line L11 (-10.15, 8.7013) -> (-9.15, 8.7013)
  line L12 (9.15, -8.7012) -> (10.15, -8.7012)
  line L13 (10.15, -8.7012) -> (10.15, -3.7012)
  line L14 (10.15, -3.7012) -> (9.15, -3.7012)
  dimension "d75" = 5
  dimension "d76" = 5
  dimension "d79" = 1
  dimension "d80" = 5
  dimension "d81" = 1
  dimension "d82" = 5
  dimension "d147" = 15.3512
  dimension "d148" = 21.5441
  dimension "d149" = 14.1416
  constraint coincident L4.start A0.centre
  constraint parallel L5 L6
  constraint parallel L7 L8
  constraint horizontal L9
  constraint vertical L10
  constraint horizontal L11
  constraint horizontal L12
  constraint vertical L13
  constraint horizontal L14
  constraint tangent L7 A1
  constraint tangent L8 A1
  constraint tangent L6 A0
  constraint tangent L5 A0
  constraint coincident L1 L7.end
  constraint coincident L1 L8.start
  constraint coincident L3 L5.end
  constraint coincident L3 L6.start
  constraint equal L5 L7
  measures "d75" diameter of A1
  measures "d76" diameter of A0
  measures "d79" distance of L7.end L9.end
  measures "d80" distance of L7.end L8.start
  measures "d81" distance of L6.start L12.end
  measures "d82" distance of L6.start L5.end
  measures "d147" distance of L1 L4
  measures "d148" distance of L2 L7
  measures "d149" distance of L2 L5
extrude "Extrude15" add sketch "Sketch6" along normal blind 12.45 contours L3 L12 L13 L14 | L3 L5 L6 A0 | L1 L7 L8 A1 | L1 L9 L10 L11
extrude "Extrude16" add 1 faces at (-2.0372, -23.65, 0.4401) along direction (0, 1, 0) blind 2
extrude "Extrude17" add 1 faces at (1.7037, 23.65, 0.4415) along direction (0, -1, 0) blind 2
equation "d45 = ( 4.3 / 2 ) * 1 mm"
equation "d46 = ( 4.3 / 2 ) * 1 mm"
equation "d53 = ( 4.3 / 2 ) * 1 mm"
equation "d54 = ( 4.3 / 2 ) * 1 mm"
equation "d55 = ( 4.3 / 2 ) * 1 mm"
equation "d77 = 5.00 mm + 7.45 mm"

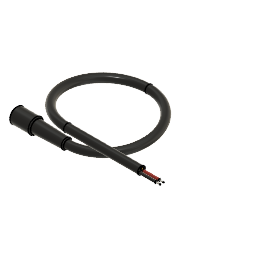
design "PE2 - 3-Pin Male Waterproof Connector (cut, coiled)"
Autodesk Fusion 360 part; units mm, degrees
sketch "Sketch1" plane through (0, 0, 0) normal (1, 0, 0) x (0, 1, 0)
  circle A0 centre (0, 0) radius 3.683
  circle A1 centre (0, 0) radius 3.175
  dimension "d1" = 7.366
  dimension "d2" = 6.35
  constraint coincident A0.centre A1.centre
  constraint concentric A0 A1
  measures "d1" diameter of A0
  measures "d2" diameter of A1
extrude "Extrude1" add sketch "Sketch1" along normal blind 10 contours A0 | A1 makes body 1
extrude "Extrude2" cut sketch "Sketch1" along normal blind 8 contours A1 bodies 1
sketch "Sketch2" plane through (0, 0, 0) normal (0, 1, 0) x (1, 0, 0)
  line L0 (10, 0) -> (10, -3)
  line L1 (10, -3) -> (25, -2.5)
  line L2 (25, -2.5) -> (25, 0)
  line L3 (25, 0) -> (10, 0)
  dimension "d7" = 3
  dimension "d46" = 15
  dimension "d47" = 88.091
  dimension "d48" = 10
  constraint vertical L0
  constraint vertical L2
  constraint perpendicular L0 L3
  constraint horizontal origin L0.start
  measures "d7" distance of L0.start L0.end
  measures "d46" distance of L0 L2
  measures "d47" angle of L0 L1
  measures "d48" distance of origin L0
revolve "Revolve1" add sketch "Sketch2" angle 360 about axis through (1.75, 0, 0) along (1, 0, 0) bodies 1
fillet "Fillet1" radius 0.5 3 edges at (0, -3.4338, -1.3318) (10, -3.4338, -1.3318) (25, -0.904, -2.3308) on bodies 1
sketch "Sketch4" plane through (8, 0, 0) normal (1, 0, 0) x (0, 1, 0)
  line L0 (0, 1.5) -> (-1.299, -0.75) construction
  line L1 (-1.299, -0.75) -> (1.299, -0.75) construction
  line L2 (1.299, -0.75) -> (0, 1.5) construction
  circle A0 centre (0, 1.5) radius 0.5
  circle A1 centre (-1.299, -0.75) radius 0.5
  circle A2 centre (1.299, -0.75) radius 0.5
  dimension "d15" = 1.5
  dimension "d16" = 1
  dimension "d17" = 1
  dimension "d18" = 1
  constraint coincident L0.start L2.end
  constraint coincident L0.end L1.start
  constraint coincident L1.end L2.start
  constraint horizontal L1
  measures "d15" distance of L0.start origin
  measures "d16" diameter of A0
  measures "d17" diameter of A1
  measures "d18" diameter of A2
extrude "Extrude4" add sketch "Sketch4" against normal blind 8 separate body makes body 2 at (2.6667, 0.4975, 1.4502) makes body 3 at (2.6667, 1.7966, -0.7998) makes body 4 at (2.6667, -0.8015, -0.7998)
fillet "Fillet2" radius 0.1 3 edges at (0, -0.4662, 1.6808) (0, 0.8329, -0.5692) (0, -1.7652, -0.5692) on bodies 2 3 4
sketch "Sketch3" plane through (25, 0, 0) normal (1, 0, 0) x (0, 1, 0)
  circle A0 centre (0, 0) radius 1.905
  circle A1 centre (0, 0) radius 2.0164
  dimension "d9" = 3.81
  constraint coincident A0.centre A1.centre
  measures "d9" diameter of A0
sketch "Sketch5" plane through (0, 0, 0) normal (0, 0, 1) x (1, 0, 0)
  arc A0 through (25, 0, 0) (45, 19.9239, 1.7431) (25, 39.8478, 3.4862)
  arc A1 through (25, 39.8478, 3.4862) (5, 19.9239, 5.2293) (25, 0, 6.9725)
  dimension "d42" = 40
  dimension "d49" = 3.4862
  dimension "d50" = 6.9725
sweep "Sweep1" add profiles "Sketch3" path "Sketch5" along A0 A1 section 1 contours A0 bodies 1
extrude "Extrude5" add 1 faces at (25, -0.7992, 7.2336) along direction (1, 0, 0) blind 36.2 on bodies 1 bodies 1
sketch "Sketch6" plane through (61.2, 0, 0) normal (1, 0, 0) x (0, 1, 0)
  line L0 (0, 7.9725) -> (-0.866, 6.4725) construction
  line L1 (-0.866, 6.4725) -> (0.866, 6.4725) construction
  line L2 (0.866, 6.4725) -> (0, 7.9725) construction
  circle A0 centre (0, 7.9725) radius 0.625
  circle A1 centre (0.866, 6.4725) radius 0.625
  circle A2 centre (-0.866, 6.4725) radius 0.625
  circle A3 centre (0, 6.9725) radius 1.905
  point P0 (0, 6.9725)
  dimension "d31" = 1
  dimension "d32" = 1.25
  dimension "d33" = 1.25
  dimension "d34" = 1.25
  constraint coincident L0.start L2.end
  constraint coincident L1.end L2.start
  constraint coincident L0.end L1.start
  constraint coincident P0 A3.centre
  constraint vertical L0.start P0
  measures "d31" distance of L0.start P0
  measures "d32" diameter of A0
  measures "d33" diameter of A1
  measures "d34" diameter of A2
extrude "Extrude6" add sketch "Sketch6" along normal blind 8 separate body contours A1 | A2 makes body 5 at (63.8667, -0.2441, 6.4102) makes body 6 at (63.8667, 1.4879, 6.4102)
sketch "Sketch7" plane through (69.2, 0, 0) normal (1, 0, 0) x (0, 1, 0)
  circle A0 centre (0, 7.9725) radius 0.375
  circle A1 centre (-0.866, 6.4725) radius 0.625
  circle A2 centre (0.866, 6.4725) radius 0.625
  dimension "d43" = 0.75
  dimension "d51" = 1.5
  dimension "d52" = 0.866
  measures "d43" diameter of A0
  measures "d51" vertical distance of A0.centre A1.centre
  measures "d52" horizontal distance of A0.centre A1.centre
sketch "Sketch8" plane through (69.2, 0, 0) normal (1, 0, 0) x (0, 1, 0)
  circle A0 centre (0.866, 6.4725) radius 0.625
  circle A1 centre (0.866, 6.4725) radius 0.375
  dimension "d37" = 0.75
  constraint concentric A0 A1
  measures "d37" diameter of A1
sketch "Sketch9" plane through (69.2, 0, 0) normal (1, 0, 0) x (0, 1, 0)
  circle A0 centre (-0.866, 6.4725) radius 0.625
  circle A1 centre (-0.866, 6.4725) radius 0.375
  dimension "d38" = 0.75
  constraint concentric A0 A1
  measures "d38" diameter of A1
extrude "Extrude7" add sketch "Sketch8" sketch "Sketch9" along normal blind 2 separate body contours A1 of sketch 2 contours A1 makes body 7 at (69.8667, 1.2392, 6.4351) makes body 8 at (69.8667, -0.4929, 6.4351)
extrude "Extrude8" add sketch "Sketch6" along normal blind 0.5 separate body contours A0 makes body 9
